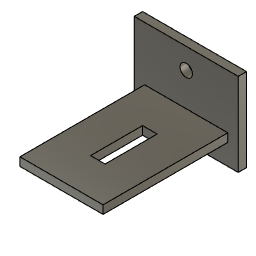
Holder kamere (Autodesk Fusion 360 design; units mm, degrees)
Autodesk Fusion 360 part; units mm, degrees
sketch "Sketch1" plane through (0, 0, 0) normal (0, 1, 0) x (1, 0, 0)
  line L0 (25, 20) -> (-25, 20)
  line L1 (-25, 20) -> (-25, -20)
  line L2 (-25, -20) -> (25, -20)
  line L3 (25, -20) -> (25, 20)
  circle A0 centre (0, -10) radius 3
  line L4 (0, 10) -> (-7.5, 10)
  line L5 (-7.5, 10) -> (-7.5, 6)
  line L6 (-7.5, 6) -> (7.5, 6)
  line L7 (7.5, 6) -> (7.5, 10)
  line L8 (7.5, 10) -> (0, 10)
  dimension "d1" = 50
  dimension "d2" = 40
  dimension "d3" = 6
  dimension "d4" = 7.5
  dimension "d5" = 4
  dimension "d6" = 15
  constraint horizontal L0
  constraint perpendicular L0 L1
  constraint parallel L0 L2
  constraint parallel L1 L3
  constraint perpendicular L4 L5
  constraint perpendicular L5 L6
  constraint perpendicular L6 L7
  measures "d1" distance of L1.end L2.end
  measures "d2" distance of L0.end L1.end
  measures "d3" diameter of A0
  measures "d4" distance of L4.start L4.end
  measures "d5" distance of L4.end L5.end
  measures "d6" distance of L5.end L6.end
extrude "Extrude1" add sketch "Sketch1" along normal blind 4 makes body 1
sketch "Sketch2" plane through (0, 0, 0) normal (0, 0, 1) x (1, 0, 0)
  line L0 (170, -30) -> (130, -30)
  line L1 (130, -30) -> (130, 30)
  line L2 (170, 30) -> (170, -30)
  line L3 (170, -30) -> (130, 30) construction
  line L4 (130, -30) -> (170, 30) construction
  line L5 (153.5, -12.5) -> (146.5, -12.5)
  line L6 (146.5, -12.5) -> (146.5, 12.5)
  line L7 (146.5, 12.5) -> (153.5, 12.5)
  line L8 (153.5, 12.5) -> (153.5, -12.5)
  line L9 (153.5, -12.5) -> (146.5, 12.5) construction
  line L10 (146.5, -12.5) -> (153.5, 12.5) construction
  line L11 (142.5, 30) -> (142.5, 34)
  line L12 (142.5, 34) -> (157.5, 34)
  line L13 (157.5, 34) -> (157.5, 30)
  line L14 (130, 30) -> (142.5, 30)
  line L15 (157.5, 30) -> (170, 30)
  point P0 (150, 0)
  point P1 (150, 0)
  dimension "d9" = 40
  dimension "d10" = 60
  dimension "d11" = 7
  dimension "d12" = 25
  dimension "d14" = 4
  dimension "d15" = 15
  constraint horizontal L0
  constraint perpendicular L0 L1
  constraint parallel L0 L14
  constraint parallel L1 L2
  constraint coincident L3 P1
  constraint coincident L4 P1
  constraint horizontal L5
  constraint perpendicular L5 L6
  constraint parallel L5 L7
  constraint parallel L6 L8
  constraint coincident L9 P1
  constraint coincident L10 P1
  constraint coincident P1 P0
  constraint perpendicular L11 L14
  constraint perpendicular L11 L12
  constraint coincident L13.end L14
  constraint perpendicular L13 L14
  constraint collinear L14 L15
  measures "d9" distance of L1.end L2.start
  measures "d10" distance of L0.end L1.end
  measures "d11" distance of L6.end L7.end
  measures "d12" distance of L5.end L6.end
  measures "d14" distance of L11.start L11.end
  measures "d15" distance of L11.end L12.end
extrude "Extrude2" add sketch "Sketch2" along normal blind 4 separate body makes body 2
copy_body "Body->Comp1" bodies 2 removing the originals makes body 3 in component "Component"
component "Component" placed x (1, 0, 0) y (0, 1, 0) z (0, 0, 1) at (-150, -30, -10)
